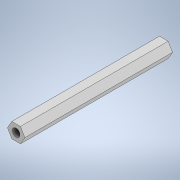
# Autodesk Inventor part: standoff_kicker
Saved by Autodesk Inventor 2020 (Build 240168000, 168)
## iProperties
Created: 2019-08-28
Part Number: standoff_kicker
Material: Generic
Document SubType Name: Modeling
Designer: Felipe
Density: 1 g/cm^3
Appearance: Default
Author: Felipe
Autodesk Inventor part; units mm, degrees
ref_plane "YZ Plane" through (0, 0, 0) normal (1, 0, 0) x (0, 1, 0)
ref_plane "XZ Plane" through (0, 0, 0) normal (0, 1, 0) x (-1, 0, 0)
sketch "Sketch1" plane through (0, 0, 0) normal (0, 0, 1) x (1, 0, 0)
  line L0 (1.5877, 2.75) -> (3.1754, 0)
  line L1 (3.1754, 0) -> (1.5877, -2.75)
  line L2 (1.5877, -2.75) -> (-1.5877, -2.75)
  line L3 (-1.5877, -2.75) -> (-3.1754, 0)
  line L4 (-3.1754, 0) -> (-1.5877, 2.75)
  line L5 (-1.5877, 2.75) -> (1.5877, 2.75)
  point P0 (0, 0)
  point P1 (0, 0)
  dimension "d0" = 5.5
  constraints: 12 end point, 1 coincident, 13 other
  measures "d0" distance between parallel lines of L2 L5
extrude "Extrusion1" add sketch "Sketch1" along normal blind 54
sketch "Sketch2" plane through (0, 0, 0) normal (0, 0, -1) x (-1, 0, 0)
  line L0 (-1.5877, 2.75) -> (1.5877, 2.75) projected
  line L1 (-3.1754, 0) -> (-1.5877, 2.75) projected
  line L2 (-1.5877, -2.75) -> (-3.1754, 0) projected
  line L3 (1.5877, -2.75) -> (-1.5877, -2.75) projected
  line L4 (3.1754, 0) -> (1.5877, -2.75) projected
  line L5 (1.5877, 2.75) -> (3.1754, 0) projected
  point P0 (0, 0)
  point P1 (0, 0)
  constraints: 1 coincident
hole "Hole1" at (0, 0, 0) direction (0, 0, 1) diameter 2.85 depth 10.4 thread size "M3.5x0.6" class "6H" standard "ISO Metric profile"
ref_plane "Work Plane1" through (0, 0, 27) normal (0, 0, -1) x (-1, 0, 0)
mirror "Mirror1" about plane through (0, 0, 27) normal (0, 0, -1) of "Hole1"
body "Solid1"
